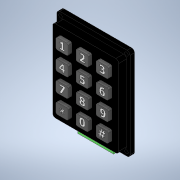
# Autodesk Inventor part: 3x4 Keypad
Saved by Autodesk Inventor 2020.2 (Build 242310000, 310)
## iProperties
Created: 2020-04-19
Part Number: 3x4 Keypad
Material: Generic
Document SubType Name: Modeling
Designer: Hayder_PC
Density: 1 g/cm^3
Appearance: Default
Author: Hayder_PC
Autodesk Inventor part; units mm, degrees
ref_plane "YZ Plane" through (0, 0, 0) normal (1, 0, 0) x (0, 1, 0)
ref_plane "XZ Plane" through (0, 0, 0) normal (0, 1, 0) x (-1, 0, 0)
sketch "Sketch1" plane through (0, 0, 0) normal (0, 0, 1) x (1, 0, 0)
  line L0 (-23.5, -32) -> (23.5, -32)
  line L1 (25.5, -30) -> (25.5, 30)
  line L2 (23.5, 32) -> (-23.5, 32)
  line L3 (-25.5, 30) -> (-25.5, -30)
  line L4 (-25.5, -32) -> (25.5, 32) construction
  line L5 (25.5, -32) -> (-25.5, 32) construction
  arc A0 (-23.5, 32) -> (-25.5, 30) centre (-23.5, 30) ccw
  arc A1 (25.5, 30) -> (23.5, 32) centre (23.5, 30) ccw
  arc A2 (23.5, -32) -> (25.5, -30) centre (23.5, -30) ccw
  arc A3 (-25.5, -30) -> (-23.5, -32) centre (-23.5, -30) ccw
  point P0 (0, 0)
  point P1 (-23, 29.5)
  point P2 (23, 29.5)
  point P3 (23, -29.5)
  point P4 (-23, -29.5)
  dimension "d0" = 64
  dimension "d1" = 51
  dimension "d7" = 2
  dimension "d26" = 2.5
  dimension "d27" = 2.5
  dimension "d28" = 46
  dimension "d29" = 59
  constraints: 12 end point, 8 point on circle, 8 point on line, 8 tangent, 4 centre point, 3 equal radius, 2 midpoint, 2 parallel, 2 vertical alignment, 1 horizontal, 1 horizontal alignment, 1 perpendicular
  measures "d0" distance of L5.start L4.end
  measures "d1" distance of L4.end L5.end
  measures "d7" radius of A0
  measures "d26" distance from line of L3 point (-23, 29.5)
  measures "d27" distance from line of L2 point (-23, 29.5)
  measures "d28" distance of point (23, 29.5) point (-23, 29.5)
  measures "d29" distance of point (23, -29.5) point (23, 29.5)
extrude "Extrusion1" add sketch "Sketch1" along normal blind 3.1
sketch "Sketch2" plane through (0, 0, 3.1) normal (0, 0, 1) x (1, 0, 0)
  line L0 (-23.5, -32) -> (23.5, -32) projected
  line L1 (25.5, -30) -> (25.5, 30) projected
  line L2 (23.5, 32) -> (-23.5, 32) projected
  line L3 (-25.5, 30) -> (-25.5, -30) projected
  line L4 (-21, -28.5) -> (21, -28.5)
  line L5 (23, -26.5) -> (23, 26.5)
  line L6 (21, 28.5) -> (-21, 28.5)
  line L7 (-23, 26.5) -> (-23, -26.5)
  line L8 (-23, -28.5) -> (23, 28.5) construction
  line L9 (23, -28.5) -> (-23, 28.5) construction
  arc A0 (-21, 28.5) -> (-23, 26.5) centre (-21, 26.5) ccw
  arc A1 (23, 26.5) -> (21, 28.5) centre (21, 26.5) ccw
  arc A2 (-23, -26.5) -> (-21, -28.5) centre (-21, -26.5) ccw
  arc A3 (21, -28.5) -> (23, -26.5) centre (21, -26.5) ccw
  arc A4 (-25.5, -30) -> (-23.5, -32) centre (-23.5, -30) ccw projected
  arc A5 (23.5, -32) -> (25.5, -30) centre (23.5, -30) ccw projected
  arc A6 (25.5, 30) -> (23.5, 32) centre (23.5, 30) ccw projected
  arc A7 (-23.5, 32) -> (-25.5, 30) centre (-23.5, 30) ccw projected
  point P0 (0, 0)
  dimension "d4" = 46
  dimension "d5" = 57
  dimension "d6" = 2
  constraints: 12 end point, 8 point on circle, 8 point on line, 8 tangent, 4 centre point, 3 equal radius, 2 midpoint, 2 parallel, 1 horizontal, 1 perpendicular
  measures "d4" distance of L8.end L9.end
  measures "d5" distance of L9.start L8.end
  measures "d6" radius of A0
extrude "Extrusion2" add sketch "Sketch2" along normal blind 5.4 contours A2 L7 A0 L6 A1 L5 A3 L4
sketch "Sketch3" plane through (0, 0, 8.5) normal (0, 0, 1) x (1, 0, 0)
  arc A0 (21, -28.5) -> (23, -26.5) centre (21, -26.5) ccw projected
  line L0 (23, -26.5) -> (23, 26.5) projected
  arc A1 (23, 26.5) -> (21, 28.5) centre (21, 26.5) ccw projected
  line L1 (21, 28.5) -> (-21, 28.5) projected
  arc A2 (-21, 28.5) -> (-23, 26.5) centre (-21, 26.5) ccw projected
  line L2 (-23, 26.5) -> (-23, -26.5) projected
  arc A3 (-23, -26.5) -> (-21, -28.5) centre (-21, -26.5) ccw projected
  line L3 (-21, -28.5) -> (21, -28.5) projected
  line L4 (10.75, 15.75) -> (17.25, 15.75)
  line L5 (18.25, 16.75) -> (18.25, 22.25)
  line L6 (17.25, 23.25) -> (10.75, 23.25)
  line L7 (9.75, 22.25) -> (9.75, 16.75)
  line L8 (9.75, 15.75) -> (18.25, 23.25) construction
  line L9 (18.25, 15.75) -> (9.75, 23.25) construction
  arc A4 (10.75, 23.25) -> (9.75, 22.25) centre (10.75, 22.25) ccw
  arc A5 (18.25, 22.25) -> (17.25, 23.25) centre (17.25, 22.25) ccw
  arc A6 (17.25, 15.75) -> (18.25, 16.75) centre (17.25, 16.75) ccw
  arc A7 (9.75, 16.75) -> (10.75, 15.75) centre (10.75, 16.75) ccw
  line L10 (-4.25, 22.25) -> (-4.25, 16.75)
  arc A8 (-4.25, 16.75) -> (-3.25, 15.75) centre (-3.25, 16.75) ccw
  arc A9 (-3.25, 23.25) -> (-4.25, 22.25) centre (-3.25, 22.25) ccw
  line L11 (-3.25, 15.75) -> (3.25, 15.75)
  line L12 (-4.25, 15.75) -> (4.25, 23.25) construction
  line L13 (4.25, 15.75) -> (-4.25, 23.25) construction
  arc A10 (3.25, 15.75) -> (4.25, 16.75) centre (3.25, 16.75) ccw
  line L14 (4.25, 16.75) -> (4.25, 22.25)
  line L15 (3.25, 23.25) -> (-3.25, 23.25)
  arc A11 (4.25, 22.25) -> (3.25, 23.25) centre (3.25, 22.25) ccw
  line L16 (-18.25, 22.25) -> (-18.25, 16.75)
  arc A12 (-18.25, 16.75) -> (-17.25, 15.75) centre (-17.25, 16.75) ccw
  arc A13 (-17.25, 23.25) -> (-18.25, 22.25) centre (-17.25, 22.25) ccw
  line L17 (-17.25, 15.75) -> (-10.75, 15.75)
  line L18 (-18.25, 15.75) -> (-9.75, 23.25) construction
  line L19 (-9.75, 15.75) -> (-18.25, 23.25) construction
  arc A14 (-10.75, 15.75) -> (-9.75, 16.75) centre (-10.75, 16.75) ccw
  line L20 (-9.75, 16.75) -> (-9.75, 22.25)
  line L21 (-10.75, 23.25) -> (-17.25, 23.25)
  arc A15 (-9.75, 22.25) -> (-10.75, 23.25) centre (-10.75, 22.25) ccw
  line L22 (9.75, 9.25) -> (9.75, 3.75)
  arc A16 (9.75, 3.75) -> (10.75, 2.75) centre (10.75, 3.75) ccw
  arc A17 (10.75, 10.25) -> (9.75, 9.25) centre (10.75, 9.25) ccw
  line L23 (10.75, 2.75) -> (17.25, 2.75)
  line L24 (9.75, 2.75) -> (18.25, 10.25) construction
  line L25 (18.25, 2.75) -> (9.75, 10.25) construction
  arc A18 (17.25, 2.75) -> (18.25, 3.75) centre (17.25, 3.75) ccw
  line L26 (18.25, 3.75) -> (18.25, 9.25)
  line L27 (17.25, 10.25) -> (10.75, 10.25)
  arc A19 (18.25, 9.25) -> (17.25, 10.25) centre (17.25, 9.25) ccw
  line L28 (-4.25, 9.25) -> (-4.25, 3.75)
  arc A20 (-4.25, 3.75) -> (-3.25, 2.75) centre (-3.25, 3.75) ccw
  arc A21 (-3.25, 10.25) -> (-4.25, 9.25) centre (-3.25, 9.25) ccw
  line L29 (-3.25, 2.75) -> (3.25, 2.75)
  line L30 (-4.25, 2.75) -> (4.25, 10.25) construction
  line L31 (4.25, 2.75) -> (-4.25, 10.25) construction
  arc A22 (3.25, 2.75) -> (4.25, 3.75) centre (3.25, 3.75) ccw
  line L32 (4.25, 3.75) -> (4.25, 9.25)
  line L33 (3.25, 10.25) -> (-3.25, 10.25)
  arc A23 (4.25, 9.25) -> (3.25, 10.25) centre (3.25, 9.25) ccw
  line L34 (-18.25, 9.25) -> (-18.25, 3.75)
  arc A24 (-18.25, 3.75) -> (-17.25, 2.75) centre (-17.25, 3.75) ccw
  arc A25 (-17.25, 10.25) -> (-18.25, 9.25) centre (-17.25, 9.25) ccw
  line L35 (-17.25, 2.75) -> (-10.75, 2.75)
  line L36 (-18.25, 2.75) -> (-9.75, 10.25) construction
  line L37 (-9.75, 2.75) -> (-18.25, 10.25) construction
  arc A26 (-10.75, 2.75) -> (-9.75, 3.75) centre (-10.75, 3.75) ccw
  line L38 (-9.75, 3.75) -> (-9.75, 9.25)
  line L39 (-10.75, 10.25) -> (-17.25, 10.25)
  arc A27 (-9.75, 9.25) -> (-10.75, 10.25) centre (-10.75, 9.25) ccw
  line L40 (9.75, -3.75) -> (9.75, -9.25)
  arc A28 (9.75, -9.25) -> (10.75, -10.25) centre (10.75, -9.25) ccw
  arc A29 (10.75, -2.75) -> (9.75, -3.75) centre (10.75, -3.75) ccw
  line L41 (10.75, -10.25) -> (17.25, -10.25)
  line L42 (9.75, -10.25) -> (18.25, -2.75) construction
  line L43 (18.25, -10.25) -> (9.75, -2.75) construction
  arc A30 (17.25, -10.25) -> (18.25, -9.25) centre (17.25, -9.25) ccw
  line L44 (18.25, -9.25) -> (18.25, -3.75)
  line L45 (17.25, -2.75) -> (10.75, -2.75)
  arc A31 (18.25, -3.75) -> (17.25, -2.75) centre (17.25, -3.75) ccw
  line L46 (-4.25, -3.75) -> (-4.25, -9.25)
  arc A32 (-4.25, -9.25) -> (-3.25, -10.25) centre (-3.25, -9.25) ccw
  arc A33 (-3.25, -2.75) -> (-4.25, -3.75) centre (-3.25, -3.75) ccw
  line L47 (-3.25, -10.25) -> (3.25, -10.25)
  line L48 (-4.25, -10.25) -> (4.25, -2.75) construction
  line L49 (4.25, -10.25) -> (-4.25, -2.75) construction
  arc A34 (3.25, -10.25) -> (4.25, -9.25) centre (3.25, -9.25) ccw
  line L50 (4.25, -9.25) -> (4.25, -3.75)
  line L51 (3.25, -2.75) -> (-3.25, -2.75)
  arc A35 (4.25, -3.75) -> (3.25, -2.75) centre (3.25, -3.75) ccw
  line L52 (-18.25, -3.75) -> (-18.25, -9.25)
  arc A36 (-18.25, -9.25) -> (-17.25, -10.25) centre (-17.25, -9.25) ccw
  arc A37 (-17.25, -2.75) -> (-18.25, -3.75) centre (-17.25, -3.75) ccw
  line L53 (-17.25, -10.25) -> (-10.75, -10.25)
  line L54 (-18.25, -10.25) -> (-9.75, -2.75) construction
  line L55 (-9.75, -10.25) -> (-18.25, -2.75) construction
  arc A38 (-10.75, -10.25) -> (-9.75, -9.25) centre (-10.75, -9.25) ccw
  line L56 (-9.75, -9.25) -> (-9.75, -3.75)
  line L57 (-10.75, -2.75) -> (-17.25, -2.75)
  arc A39 (-9.75, -3.75) -> (-10.75, -2.75) centre (-10.75, -3.75) ccw
  line L58 (9.75, -16.75) -> (9.75, -22.25)
  arc A40 (9.75, -22.25) -> (10.75, -23.25) centre (10.75, -22.25) ccw
  arc A41 (10.75, -15.75) -> (9.75, -16.75) centre (10.75, -16.75) ccw
  line L59 (10.75, -23.25) -> (17.25, -23.25)
  line L60 (9.75, -23.25) -> (18.25, -15.75) construction
  line L61 (18.25, -23.25) -> (9.75, -15.75) construction
  arc A42 (17.25, -23.25) -> (18.25, -22.25) centre (17.25, -22.25) ccw
  line L62 (18.25, -22.25) -> (18.25, -16.75)
  line L63 (17.25, -15.75) -> (10.75, -15.75)
  arc A43 (18.25, -16.75) -> (17.25, -15.75) centre (17.25, -16.75) ccw
  line L64 (-4.25, -16.75) -> (-4.25, -22.25)
  arc A44 (-4.25, -22.25) -> (-3.25, -23.25) centre (-3.25, -22.25) ccw
  arc A45 (-3.25, -15.75) -> (-4.25, -16.75) centre (-3.25, -16.75) ccw
  line L65 (-3.25, -23.25) -> (3.25, -23.25)
  line L66 (-4.25, -23.25) -> (4.25, -15.75) construction
  line L67 (4.25, -23.25) -> (-4.25, -15.75) construction
  arc A46 (3.25, -23.25) -> (4.25, -22.25) centre (3.25, -22.25) ccw
  line L68 (4.25, -22.25) -> (4.25, -16.75)
  line L69 (3.25, -15.75) -> (-3.25, -15.75)
  arc A47 (4.25, -16.75) -> (3.25, -15.75) centre (3.25, -16.75) ccw
  line L70 (-18.25, -16.75) -> (-18.25, -22.25)
  arc A48 (-18.25, -22.25) -> (-17.25, -23.25) centre (-17.25, -22.25) ccw
  arc A49 (-17.25, -15.75) -> (-18.25, -16.75) centre (-17.25, -16.75) ccw
  line L71 (-17.25, -23.25) -> (-10.75, -23.25)
  line L72 (-18.25, -23.25) -> (-9.75, -15.75) construction
  line L73 (-9.75, -23.25) -> (-18.25, -15.75) construction
  arc A50 (-10.75, -23.25) -> (-9.75, -22.25) centre (-10.75, -22.25) ccw
  line L74 (-9.75, -22.25) -> (-9.75, -16.75)
  line L75 (-10.75, -15.75) -> (-17.25, -15.75)
  arc A51 (-9.75, -16.75) -> (-10.75, -15.75) centre (-10.75, -16.75) ccw
  point P0 (0, 0)
  point P1 (14, 19.5)
  point P2 (0, 19.5)
  point P3 (-14, 19.5)
  point P4 (14, 6.5)
  point P5 (0, 6.5)
  point P6 (-14, 6.5)
  point P7 (14, -6.5)
  point P8 (0, -6.5)
  point P9 (-14, -6.5)
  point P10 (14, -19.5)
  point P11 (0, -19.5)
  point P12 (-14, -19.5)
  dimension "d10" = 8.5
  dimension "d11" = 7.5
  dimension "d12" = 1
  dimension "d15" = 9
  dimension "d18" = 14
  dimension "d21" = 13
  constraints: 144 end point, 96 point on circle, 96 point on line, 48 centre point, 24 midpoint, 8 tangent, 3 equal radius, 2 collinear, 2 horizontal, 2 parallel, 1 perpendicular, 1 vertical, 295 other
  measures "d10" distance of L8.end L9.end
  measures "d11" distance of L9.start L8.end
  measures "d12" radius of A4
  measures "d15" distance from line of L0 point (14, 19.5)
  measures "d18" distance of L8.start L12.start
  measures "d21" distance of L8.start L24.start
extrude "Extrusion3" add sketch "Sketch3" along normal blind 2.5 contours A7 L7 A4 L6 A5 L5 A6 L4 | A9 L15 A11 L14 A10 L11 A8 L10 | A13 L21 A15 L20 A14 L17 A12 L16 | A17 L27 A19 L26 A18 L23 A16 L22 | A21 L33 A23 L32 A22 L29 A20 L28 | A25 L39 A27 L38 A26 L35 A24 L34 | A29 L45 A31 L44 A30 L41 A28 L40 | A33 L51 A35 L50 A34 L47 A32 L46 | A37 L57 A39 L56 A38 L53 A36 L52 | A41 L63 A43 L62 A42 L59 A40 L58 | A45 L69 A47 L68 A46 L65 A44 L64 | A49 L75 A51 L74 A50 L71 A48 L70
sketch "Sketch4" plane through (0, 0, 3.1) normal (0, 0, 1) x (1, 0, 0)
  line L0 (-21, 28.5) -> (21, 28.5) projected
  arc A0 (23, 26.5) -> (21, 28.5) centre (21, 26.5) ccw projected
  line L1 (23, 26.5) -> (23, -26.5) projected
  arc A1 (21, -28.5) -> (23, -26.5) centre (21, -26.5) ccw projected
  line L2 (21, -28.5) -> (-21, -28.5) projected
  arc A2 (-23, -26.5) -> (-21, -28.5) centre (-21, -26.5) ccw projected
  line L3 (-23, -26.5) -> (-23, 26.5) projected
  arc A3 (-21, 28.5) -> (-23, 26.5) centre (-21, 26.5) ccw projected
  line L4 (-23.5, -32) -> (23.5, -32) projected
  arc A4 (23.5, -32) -> (25.5, -30) centre (23.5, -30) ccw projected
  line L5 (25.5, -30) -> (25.5, 30) projected
  arc A5 (25.5, 30) -> (23.5, 32) centre (23.5, 30) ccw projected
  line L6 (23.5, 32) -> (-23.5, 32) projected
  arc A6 (-23.5, 32) -> (-25.5, 30) centre (-23.5, 30) ccw projected
  line L7 (-25.5, 30) -> (-25.5, -30) projected
  arc A7 (-25.5, -30) -> (-23.5, -32) centre (-23.5, -30) ccw projected
  point P0 (0, 0)
  point P1 (-23, 29.5)
  point P2 (23, 29.5)
  point P3 (23, -29.5)
  point P4 (-23, -29.5)
  dimension "d30" = 2.5
  dimension "d31" = 2.5
  dimension "d32" = 46
  dimension "d33" = 59
  constraints: 2 horizontal alignment, 2 vertical alignment
  measures "d30" distance from line of L6 point (-23, 29.5)
  measures "d31" distance from line of L7 point (-23, 29.5)
  measures "d32" distance of point (23, 29.5) point (-23, 29.5)
  measures "d33" distance of point (23, -29.5) point (23, 29.5)
hole "Hole1" at (-23, 29.5, 3.1) at (23, 29.5, 3.1) at (23, -29.5, 3.1) at (-23, -29.5, 3.1) direction (0, 0, -1) diameter 2.4 end through all
ref_plane "Work Plane2" through (0, 0, 1.5) normal (0, 0, 1) x (1, 0, 0)
sketch "Sketch8" plane through (0, 0, 1.5) normal (0, 0, 1) x (1, 0, 0)
  line L0 (-23.5, -32) -> (23.5, -32) projected
  line L1 (-12.5, -32) -> (12.5, -32)
  line L2 (12.5, -32) -> (12.5, -37)
  line L3 (12.5, -37) -> (-12.5, -37)
  line L4 (-12.5, -37) -> (-12.5, -32)
  line L5 (-25.5, 30) -> (-25.5, -30) projected
  point P0 (0, 0)
  point P1 (12.5, -32)
  dimension "d60" = 25
  dimension "d61" = 5
  dimension "d62" = 13
  constraints: 8 end point, 2 parallel, 1 horizontal, 1 perpendicular, 1 point on line
  measures "d60" distance of L2.end L3.end
  measures "d61" distance of L1.end L2.end
  measures "d62" distance between parallel lines of L5 L4
extrude "Extrusion6" add sketch "Sketch8" against normal blind 1
sketch "Sketch9" plane through (0, 0, 1.5) normal (0, 0, 1) x (1, 0, 0)
  circle A0 centre (-8.75, -34.5) radius 0.5
  line L0 (-12.5, -32) -> (-12.5, -37) projected
  line L1 (-12.5, -37) -> (12.5, -37) projected
  line L2 (-8.75, -34.5) -> (7.0736, -34.5) construction
  line L3 (-6.25, -34.5) -> (9.5736, -34.5) construction
  circle A1 centre (-6.25, -34.5) radius 0.5
  line L4 (-3.75, -34.5) -> (12.0736, -34.5) construction
  circle A2 centre (-3.75, -34.5) radius 0.5
  line L5 (-1.25, -34.5) -> (14.5736, -34.5) construction
  circle A3 centre (-1.25, -34.5) radius 0.5
  line L6 (1.25, -34.5) -> (17.0736, -34.5) construction
  circle A4 centre (1.25, -34.5) radius 0.5
  line L7 (3.75, -34.5) -> (19.5736, -34.5) construction
  circle A5 centre (3.75, -34.5) radius 0.5
  line L8 (6.25, -34.5) -> (22.0736, -34.5) construction
  circle A6 centre (6.25, -34.5) radius 0.5
  line L9 (8.75, -34.5) -> (24.5736, -34.5) construction
  circle A7 centre (8.75, -34.5) radius 0.5
  point P0 (0, 0)
  dimension "d65" = 1
  dimension "d66" = 3.75
  dimension "d67" = 2.5
  dimension "d70" = 2.5
  constraints: 16 end point, 8 centre point, 2 horizontal, 1 collinear, 27 other
  measures "d65" diameter of A0
  measures "d66" distance from line of L0 L2.start
  measures "d67" distance from line of L1 L2.start
  measures "d70" distance of L2.start L3.start
extrude "Extrusion7" cut sketch "Sketch9" against normal blind 1
sketch "Sketch11" plane through (0, 0, 11) normal (0, 0, 1) x (1, 0, 0)
  line L0 (-16.2137, 22.189) -> (-9.5825, 22.189) construction
  line L1 (-9.5825, 22.189) -> (-9.5825, 17.2629) construction
  line L2 (-9.5825, 17.2629) -> (-16.2137, 17.2629) construction
  line L3 (-16.2137, 17.2629) -> (-16.2137, 22.189) construction
  line L4 (-2.1702, 22.189) -> (4.461, 22.189) construction
  line L5 (4.461, 22.189) -> (4.461, 17.2629) construction
  line L6 (4.461, 17.2629) -> (-2.1702, 17.2629) construction
  line L7 (-2.1702, 17.2629) -> (-2.1702, 22.189) construction
  line L8 (11.6989, 22.189) -> (18.3301, 22.189) construction
  line L9 (18.3301, 22.189) -> (18.3301, 17.2629) construction
  line L10 (18.3301, 17.2629) -> (11.6989, 17.2629) construction
  line L11 (11.6989, 17.2629) -> (11.6989, 22.189) construction
  line L12 (-16.2137, 8.9305) -> (-9.5825, 8.9305) construction
  line L13 (-9.5825, 8.9305) -> (-9.5825, 4.0044) construction
  line L14 (-9.5825, 4.0044) -> (-16.2137, 4.0044) construction
  line L15 (-16.2137, 4.0044) -> (-16.2137, 8.9305) construction
  line L16 (-2.1702, 8.9305) -> (4.461, 8.9305) construction
  line L17 (4.461, 8.9305) -> (4.461, 4.0044) construction
  line L18 (4.461, 4.0044) -> (-2.1702, 4.0044) construction
  line L19 (-2.1702, 4.0044) -> (-2.1702, 8.9305) construction
  line L20 (11.6989, 8.9305) -> (18.3301, 8.9305) construction
  line L21 (18.3301, 8.9305) -> (18.3301, 4.0044) construction
  line L22 (18.3301, 4.0044) -> (11.6989, 4.0044) construction
  line L23 (11.6989, 4.0044) -> (11.6989, 8.9305) construction
  line L24 (-16.2137, -4.0005) -> (-9.5825, -4.0005) construction
  line L25 (-9.5825, -4.0005) -> (-9.5825, -8.9266) construction
  line L26 (-9.5825, -8.9266) -> (-16.2137, -8.9266) construction
  line L27 (-16.2137, -8.9266) -> (-16.2137, -4.0005) construction
  line L28 (-2.1702, -4.0005) -> (4.461, -4.0005) construction
  line L29 (4.461, -4.0005) -> (4.461, -8.9266) construction
  line L30 (4.461, -8.9266) -> (-2.1702, -8.9266) construction
  line L31 (-2.1702, -8.9266) -> (-2.1702, -4.0005) construction
  line L32 (12.2001, -4.0005) -> (18.8313, -4.0005) construction
  line L33 (18.8313, -4.0005) -> (18.8313, -8.9266) construction
  line L34 (18.8313, -8.9266) -> (12.2001, -8.9266) construction
  line L35 (12.2001, -8.9266) -> (12.2001, -4.0005) construction
  line L36 (10.8904, -16.8079) -> (17.5216, -16.8079) construction
  line L37 (17.5216, -16.8079) -> (17.5216, -21.734) construction
  line L38 (17.5216, -21.734) -> (10.8904, -21.734) construction
  line L39 (10.8904, -21.734) -> (10.8904, -16.8079) construction
  line L40 (-2.1702, -16.6356) -> (4.461, -16.6356) construction
  line L41 (4.461, -16.6356) -> (4.461, -21.5617) construction
  line L42 (4.461, -21.5617) -> (-2.1702, -21.5617) construction
  line L43 (-2.1702, -21.5617) -> (-2.1702, -16.6356) construction
  line L44 (-16.1103, -17.8074) -> (-9.4791, -17.8074) construction
  line L45 (-9.4791, -17.8074) -> (-9.4791, -22.7335) construction
  line L46 (-9.4791, -22.7335) -> (-16.1103, -22.7335) construction
  line L47 (-16.1103, -22.7335) -> (-16.1103, -17.8074) construction
  line L48 (-12.2551, 17.1769) -> (-15.5573, 17.1769)
  line L49 (-15.5573, 17.1769) -> (-15.5573, 18.048)
  line L50 (-15.5573, 18.048) -> (-14.5039, 18.048)
  line L51 (-14.5039, 18.048) -> (-14.5039, 20.6939)
  line L52 (-14.5039, 20.6939) -> (-15.5573, 20.6939)
  line L53 (-15.5573, 20.6939) -> (-15.5573, 21.5083)
  spline S0 degree 2 poles (-15.5573, 21.5083) (-15.3264, 21.5083) (-14.8685, 21.5691) (-14.7308, 21.6339) knots 0 0 0 1 2 2 2
  spline S1 degree 2 poles (-14.7308, 21.6339) (-14.5727, 21.7149) (-14.3944, 21.9864) (-14.3782, 22.189) knots 0 0 0 1 2 2 2
  line L54 (-14.3782, 22.189) -> (-13.2842, 22.189)
  line L55 (-13.2842, 22.189) -> (-13.2842, 18.048)
  line L56 (-13.2842, 18.048) -> (-12.2551, 18.048)
  line L57 (-12.2551, 18.048) -> (-12.2551, 17.1769)
  line L58 (2.0113, 17.0918) -> (-1.6637, 17.0918)
  line L59 (-1.6637, 17.0918) -> (-1.6637, 17.9062)
  spline S2 degree 2 poles (-1.6637, 17.9062) (-1.1978, 18.279) (-0.4522, 18.9354) (-0.1726, 19.2311) knots 0 0 0 1 2 2 2
  spline S3 degree 2 poles (-0.1726, 19.2311) (0.1961, 19.6161) (0.5243, 20.2036) (0.5243, 20.5115) knots 0 0 0 1 2 2 2
  spline S4 degree 2 poles (0.5243, 20.5115) (0.5243, 20.86) (0.1069, 21.2328) (-0.2658, 21.2328) knots 0 0 0 1 2 2 2
  spline S5 degree 2 poles (-0.2658, 21.2328) (-0.4563, 21.2328) (-0.7966, 21.1396) (-0.9709, 21.0666) knots 0 0 0 1 2 2 2
  spline S6 degree 2 poles (-0.9709, 21.0666) (-1.141, 20.9897) (-1.3842, 20.8276) (-1.4449, 20.7871) knots 0 0 0 1 2 2 2
  line L60 (-1.4449, 20.7871) -> (-1.5422, 20.7871)
  line L61 (-1.5422, 20.7871) -> (-1.5422, 21.877)
  spline S7 degree 2 poles (-1.5422, 21.877) (-1.3315, 21.9783) (-0.432, 22.189) (-0.0146, 22.189) knots 0 0 0 1 2 2 2
  spline S8 degree 2 poles (-0.0146, 22.189) (0.8768, 22.189) (1.7925, 21.3948) (1.7925, 20.6777) knots 0 0 0 1 2 2 2
  spline S9 degree 2 poles (1.7925, 20.6777) (1.7925, 20.236) (1.3752, 19.3851) (0.893, 18.8989) knots 0 0 0 1 2 2 2
  spline S10 degree 2 poles (0.893, 18.8989) (0.5891, 18.5991) (0.0178, 18.1331) (-0.1078, 18.0358) knots 0 0 0 1 2 2 2
  line L62 (-0.1078, 18.0358) -> (2.0113, 18.0358)
  line L63 (2.0113, 18.0358) -> (2.0113, 17.0918)
  line L64 (-12.3056, -20.1412) -> (-12.6501, -20.6518)
  line L65 (-12.6501, -20.6518) -> (-13.6995, -19.9387)
  line L66 (-13.6995, -19.9387) -> (-13.663, -21.1056)
  line L67 (-13.663, -21.1056) -> (-14.3356, -21.1056)
  line L68 (-14.3356, -21.1056) -> (-14.3154, -19.9711)
  line L69 (-14.3154, -19.9711) -> (-15.3405, -20.6558)
  line L70 (-15.3405, -20.6558) -> (-15.6849, -20.1372)
  line L71 (-15.6849, -20.1372) -> (-14.5261, -19.4565)
  line L72 (-14.5261, -19.4565) -> (-15.6768, -18.7677)
  line L73 (-15.6768, -18.7677) -> (-15.3405, -18.249)
  line L74 (-15.3405, -18.249) -> (-14.3154, -18.9459)
  line L75 (-14.3154, -18.9459) -> (-14.3356, -17.8074)
  line L76 (-14.3356, -17.8074) -> (-13.6671, -17.8074)
  line L77 (-13.6671, -17.8074) -> (-13.6873, -18.9459)
  line L78 (-13.6873, -18.9459) -> (-12.6501, -18.2531)
  line L79 (-12.6501, -18.2531) -> (-12.3056, -18.7717)
  line L80 (-12.3056, -18.7717) -> (-13.4685, -19.4524)
  line L81 (-13.4685, -19.4524) -> (-12.3056, -20.1412)
  spline S11 degree 2 poles (1.9465, -19.2369) (1.9465, -19.8852) (1.7398, -20.8576) (1.5089, -21.1858) knots 0 0 0 1 2 2 2
  spline S12 degree 2 poles (1.5089, -21.1858) (1.282, -21.51) (0.5486, -21.8423) (0.0218, -21.8423) knots 0 0 0 1 2 2 2
  spline S13 degree 2 poles (0.0218, -21.8423) (-0.5089, -21.8423) (-1.2383, -21.51) (-1.4692, -21.1777) knots 0 0 0 1 2 2 2
  spline S14 degree 2 poles (-1.4692, -21.1777) (-1.7002, -20.8495) (-1.9068, -19.8852) (-1.9068, -19.2369) knots 0 0 0 1 2 2 2
  spline S15 degree 2 poles (-1.9068, -19.2369) (-1.9068, -18.5724) (-1.7002, -17.6324) (-1.4652, -17.292) knots 0 0 0 1 2 2 2
  spline S16 degree 2 poles (-1.4652, -17.292) (-1.2302, -16.9598) (-0.4887, -16.6356) (0.0218, -16.6356) knots 0 0 0 1 2 2 2
  spline S17 degree 2 poles (0.0218, -16.6356) (0.5607, -16.6356) (1.282, -16.976) (1.5129, -17.3123) knots 0 0 0 1 2 2 2
  spline S18 degree 2 poles (1.5129, -17.3123) (1.7398, -17.6405) (1.9465, -18.6089) (1.9465, -19.2369) knots 0 0 0 1 2 2 2
  spline S19 degree 2 poles (0.6864, -19.2369) (0.6864, -18.309) (0.3825, -17.5594) (0.0218, -17.5594) knots 0 0 0 1 2 2 2
  spline S20 degree 2 poles (0.0218, -17.5594) (-0.3388, -17.5594) (-0.6467, -18.309) (-0.6467, -19.241) knots 0 0 0 1 2 2 2
  spline S21 degree 2 poles (-0.6467, -19.241) (-0.6467, -20.1567) (-0.3388, -20.9184) (0.0218, -20.9184) knots 0 0 0 1 2 2 2
  spline S22 degree 2 poles (0.0218, -20.9184) (0.3784, -20.9184) (0.6864, -20.1567) (0.6864, -19.2369) knots 0 0 0 1 2 2 2
  line L82 (16.1011, -18.7447) -> (15.076, -18.7447)
  line L83 (15.076, -18.7447) -> (14.8045, -19.8428)
  line L84 (14.8045, -19.8428) -> (15.7122, -19.8428)
  line L85 (15.7122, -19.8428) -> (15.7122, -20.6167)
  line L86 (15.7122, -20.6167) -> (14.606, -20.6167)
  line L87 (14.606, -20.6167) -> (14.3062, -21.8079)
  line L88 (14.3062, -21.8079) -> (13.5282, -21.8079)
  line L89 (13.5282, -21.8079) -> (13.828, -20.6167)
  line L90 (13.828, -20.6167) -> (12.965, -20.6167)
  line L91 (12.965, -20.6167) -> (12.6652, -21.8079)
  line L92 (12.6652, -21.8079) -> (11.8791, -21.8079)
  line L93 (11.8791, -21.8079) -> (12.1789, -20.6167)
  line L94 (12.1789, -20.6167) -> (11.3078, -20.6167)
  line L95 (11.3078, -20.6167) -> (11.3078, -19.8428)
  line L96 (11.3078, -19.8428) -> (12.3734, -19.8428)
  line L97 (12.3734, -19.8428) -> (12.6449, -18.7447)
  line L98 (12.6449, -18.7447) -> (11.7008, -18.7447)
  line L99 (11.7008, -18.7447) -> (11.7008, -17.9708)
  line L100 (11.7008, -17.9708) -> (12.8394, -17.9708)
  line L101 (12.8394, -17.9708) -> (13.1311, -16.8079)
  line L102 (13.1311, -16.8079) -> (13.9212, -16.8079)
  line L103 (13.9212, -16.8079) -> (13.6295, -17.9708)
  line L104 (13.6295, -17.9708) -> (14.4885, -17.9708)
  line L105 (14.4885, -17.9708) -> (14.7802, -16.8079)
  line L106 (14.7802, -16.8079) -> (15.5704, -16.8079)
  line L107 (15.5704, -16.8079) -> (15.2746, -17.9708)
  line L108 (15.2746, -17.9708) -> (16.1011, -17.9708)
  line L109 (16.1011, -17.9708) -> (16.1011, -18.7447)
  line L110 (14.3062, -18.7366) -> (13.4269, -18.7366)
  line L111 (13.4269, -18.7366) -> (13.1473, -19.8509)
  line L112 (13.1473, -19.8509) -> (14.0266, -19.8509)
  line L113 (14.0266, -19.8509) -> (14.3062, -18.7366)
  spline S23 degree 2 poles (16.2519, -6.3222) (16.2519, -6.9584) (15.9561, -8.02) (15.6442, -8.4008) knots 0 0 0 1 2 2 2
  spline S24 degree 2 poles (15.6442, -8.4008) (15.32, -8.7858) (14.3638, -9.1991) (13.6668, -9.1991) knots 0 0 0 1 2 2 2
  spline S25 degree 2 poles (13.6668, -9.1991) (13.4318, -9.1991) (12.9213, -9.1383) (12.8362, -9.114) knots 0 0 0 1 2 2 2
  line L114 (12.8362, -9.114) -> (12.8362, -8.1334)
  line L115 (12.8362, -8.1334) -> (12.9335, -8.1334)
  spline S26 degree 2 poles (12.9335, -8.1334) (13.0267, -8.182) (13.3751, -8.2874) (13.679, -8.2874) knots 0 0 0 1 2 2 2
  spline S27 degree 2 poles (13.679, -8.2874) (13.9262, -8.2874) (14.384, -8.1577) (14.5461, -8.0159) knots 0 0 0 1 2 2 2
  spline S28 degree 2 poles (14.5461, -8.0159) (14.7203, -7.866) (14.9472, -7.4243) (14.9878, -7.0921) knots 0 0 0 1 2 2 2
  spline S29 degree 2 poles (14.9878, -7.0921) (14.7203, -7.2582) (14.2584, -7.4365) (13.914, -7.4365) knots 0 0 0 1 2 2 2
  spline S30 degree 2 poles (13.914, -7.4365) (13.6587, -7.4365) (13.1847, -7.2987) (12.9902, -7.1529) knots 0 0 0 1 2 2 2
  spline S31 degree 2 poles (12.9902, -7.1529) (12.7309, -6.9543) (12.427, -6.3182) (12.427, -5.8158) knots 0 0 0 1 2 2 2
  spline S32 degree 2 poles (12.427, -5.8158) (12.427, -5.4227) (12.6944, -4.7623) (12.9375, -4.5192) knots 0 0 0 1 2 2 2
  spline S33 degree 2 poles (12.9375, -4.5192) (13.1806, -4.276) (13.8856, -4.0005) (14.3192, -4.0005) knots 0 0 0 1 2 2 2
  spline S34 degree 2 poles (14.3192, -4.0005) (14.7568, -4.0005) (15.4335, -4.2436) (15.6766, -4.4989) knots 0 0 0 1 2 2 2
  spline S35 degree 2 poles (15.6766, -4.4989) (15.9602, -4.7825) (16.2519, -5.682) (16.2519, -6.3222) knots 0 0 0 1 2 2 2
  spline S36 degree 2 poles (15.008, -6.1358) (15.008, -5.7266) (14.8702, -5.1999) (14.7446, -5.054) knots 0 0 0 1 2 2 2
  spline S37 degree 2 poles (14.7446, -5.054) (14.6596, -4.9446) (14.4408, -4.8514) (14.3151, -4.8514) knots 0 0 0 1 2 2 2
  spline S38 degree 2 poles (14.3151, -4.8514) (14.2017, -4.8514) (13.991, -4.9405) (13.8937, -5.054) knots 0 0 0 1 2 2 2
  spline S39 degree 2 poles (13.8937, -5.054) (13.8087, -5.1512) (13.6871, -5.5281) (13.6871, -5.7509) knots 0 0 0 1 2 2 2
  spline S40 degree 2 poles (13.6871, -5.7509) (13.6871, -5.994) (13.8127, -6.306) (13.9181, -6.3992) knots 0 0 0 1 2 2 2
  spline S41 degree 2 poles (13.9181, -6.3992) (14.0275, -6.4924) (14.2989, -6.5653) (14.4691, -6.5653) knots 0 0 0 1 2 2 2
  spline S42 degree 2 poles (14.4691, -6.5653) (14.6109, -6.5653) (14.9067, -6.4884) (14.9999, -6.4478) knots 0 0 0 1 2 2 2
  spline S43 degree 2 poles (14.9999, -6.4478) (14.9999, -6.4114) (15.008, -6.2736) (15.008, -6.1358) knots 0 0 0 1 2 2 2
  spline S44 degree 2 poles (1.9992, -7.7242) (1.9992, -8.0443) (1.7317, -8.5994) (1.4765, -8.802) knots 0 0 0 1 2 2 2
  spline S45 degree 2 poles (1.4765, -8.802) (1.2212, -9.0046) (0.4878, -9.2315) (0.0137, -9.2315) knots 0 0 0 1 2 2 2
  spline S46 degree 2 poles (0.0137, -9.2315) (-0.4927, -9.2315) (-1.2504, -9.0005) (-1.4936, -8.802) knots 0 0 0 1 2 2 2
  spline S47 degree 2 poles (-1.4936, -8.802) (-1.7326, -8.6034) (-1.9595, -8.0645) (-1.9595, -7.7647) knots 0 0 0 1 2 2 2
  spline S48 degree 2 poles (-1.9595, -7.7647) (-1.9595, -7.3352) (-1.4854, -6.7639) (-1.0357, -6.5735) knots 0 0 0 1 2 2 2
  line L116 (-1.0357, -6.5735) -> (-1.0357, -6.5532)
  spline S49 degree 2 poles (-1.0357, -6.5532) (-1.4773, -6.3384) (-1.8258, -5.7266) (-1.8258, -5.3498) knots 0 0 0 1 2 2 2
  spline S50 degree 2 poles (-1.8258, -5.3498) (-1.8258, -5.0743) (-1.5827, -4.5921) (-1.3436, -4.4017) knots 0 0 0 1 2 2 2
  spline S51 degree 2 poles (-1.3436, -4.4017) (-1.1127, -4.2193) (-0.4117, -4.0005) (0.0259, -4.0005) knots 0 0 0 1 2 2 2
  spline S52 degree 2 poles (0.0259, -4.0005) (0.4878, -4.0005) (1.1766, -4.1991) (1.3995, -4.3611) knots 0 0 0 1 2 2 2
  spline S53 degree 2 poles (1.3995, -4.3611) (1.6264, -4.5232) (1.8695, -4.9932) (1.8695, -5.2647) knots 0 0 0 1 2 2 2
  spline S54 degree 2 poles (1.8695, -5.2647) (1.8695, -5.6213) (1.4562, -6.1926) (1.0308, -6.3911) knots 0 0 0 1 2 2 2
  line L117 (1.0308, -6.3911) -> (1.0308, -6.4073)
  spline S55 degree 2 poles (1.0308, -6.4073) (1.5291, -6.6099) (1.9992, -7.2663) (1.9992, -7.7242) knots 0 0 0 1 2 2 2
  spline S56 degree 2 poles (0.7593, -7.7769) (0.7593, -7.5297) (0.5486, -7.2704) (0.2082, -7.1042) knots 0 0 0 1 2 2 2
  spline S57 degree 2 poles (0.2082, -7.1042) (0.111, -7.0597) (-0.2577, -6.9179) (-0.3995, -6.8571) knots 0 0 0 1 2 2 2
  spline S58 degree 2 poles (-0.3995, -6.8571) (-0.5292, -6.9867) (-0.7359, -7.3757) (-0.7359, -7.6067) knots 0 0 0 1 2 2 2
  spline S59 degree 2 poles (-0.7359, -7.6067) (-0.7359, -7.9551) (-0.2901, -8.3725) (0.0705, -8.3725) knots 0 0 0 1 2 2 2
  spline S60 degree 2 poles (0.0705, -8.3725) (0.1718, -8.3725) (0.423, -8.3076) (0.5202, -8.2428) knots 0 0 0 1 2 2 2
  spline S61 degree 2 poles (0.5202, -8.2428) (0.6296, -8.1658) (0.7593, -7.9551) (0.7593, -7.7769) knots 0 0 0 1 2 2 2
  spline S62 degree 2 poles (0.6499, -5.4106) (0.6499, -5.1553) (0.3136, -4.8514) (0.0259, -4.8514) knots 0 0 0 1 2 2 2
  spline S63 degree 2 poles (0.0259, -4.8514) (-0.2496, -4.8514) (-0.5859, -5.1269) (-0.5859, -5.3295) knots 0 0 0 1 2 2 2
  spline S64 degree 2 poles (-0.5859, -5.3295) (-0.5859, -5.5281) (-0.3833, -5.7752) (-0.1686, -5.8765) knots 0 0 0 1 2 2 2
  spline S65 degree 2 poles (-0.1686, -5.8765) (-0.0754, -5.9252) (0.1839, -6.0264) (0.3987, -6.1075) knots 0 0 0 1 2 2 2
  spline S66 degree 2 poles (0.3987, -6.1075) (0.5283, -5.9373) (0.6499, -5.6172) (0.6499, -5.4106) knots 0 0 0 1 2 2 2
  line L118 (-12.1416, -4.9932) -> (-14.2769, -9.0005)
  line L119 (-14.2769, -9.0005) -> (-15.6708, -9.0005)
  line L120 (-15.6708, -9.0005) -> (-13.4382, -4.9446)
  line L121 (-13.4382, -4.9446) -> (-15.8207, -4.9446)
  line L122 (-15.8207, -4.9446) -> (-15.8207, -4.0005)
  line L123 (-15.8207, -4.0005) -> (-12.1416, -4.0005)
  line L124 (-12.1416, -4.0005) -> (-12.1416, -4.9932)
  line L125 (-11.9714, 5.0975) -> (-12.6481, 5.0975)
  line L126 (-12.6481, 5.0975) -> (-12.6481, 3.9184)
  line L127 (-12.6481, 3.9184) -> (-13.8596, 3.9184)
  line L128 (-13.8596, 3.9184) -> (-13.8596, 5.0975)
  line L129 (-13.8596, 5.0975) -> (-16.0638, 5.0975)
  line L130 (-16.0638, 5.0975) -> (-16.0638, 6.0294)
  line L131 (-16.0638, 6.0294) -> (-13.9001, 8.9305)
  line L132 (-13.9001, 8.9305) -> (-12.6481, 8.9305)
  line L133 (-12.6481, 8.9305) -> (-12.6481, 5.997)
  line L134 (-12.6481, 5.997) -> (-11.9714, 5.997)
  line L135 (-11.9714, 5.997) -> (-11.9714, 5.0975)
  line L136 (-13.8596, 5.997) -> (-13.8596, 7.6988)
  line L137 (-13.8596, 7.6988) -> (-15.1278, 5.997)
  line L138 (-15.1278, 5.997) -> (-13.8596, 5.997)
  spline S67 degree 2 poles (1.8979, 5.6242) (1.8979, 5.2312) (1.6304, 4.5667) (1.3671, 4.3276) knots 0 0 0 1 2 2 2
  spline S68 degree 2 poles (1.3671, 4.3276) (1.1037, 4.0885) (0.3825, 3.8252) (-0.1443, 3.8252) knots 0 0 0 1 2 2 2
  spline S69 degree 2 poles (-0.1443, 3.8252) (-0.7034, 3.8292) (-1.5057, 4.0116) (-1.7691, 4.1291) knots 0 0 0 1 2 2 2
  line L139 (-1.7691, 4.1291) -> (-1.7691, 5.219)
  line L140 (-1.7691, 5.219) -> (-1.6556, 5.219)
  spline S70 degree 2 poles (-1.6556, 5.219) (-1.5584, 5.1663) (-1.3234, 5.0286) (-1.1329, 4.9556) knots 0 0 0 1 2 2 2
  spline S71 degree 2 poles (-1.1329, 4.9556) (-0.9547, 4.8868) (-0.5859, 4.7936) (-0.3631, 4.7936) knots 0 0 0 1 2 2 2
  spline S72 degree 2 poles (-0.3631, 4.7936) (-0.1686, 4.7936) (0.2852, 4.8908) (0.423, 5.0205) knots 0 0 0 1 2 2 2
  spline S73 degree 2 poles (0.423, 5.0205) (0.5243, 5.1218) (0.6377, 5.3689) (0.6377, 5.5756) knots 0 0 0 1 2 2 2
  spline S74 degree 2 poles (0.6377, 5.5756) (0.6377, 5.7539) (0.4919, 6.0051) (0.3744, 6.0821) knots 0 0 0 1 2 2 2
  spline S75 degree 2 poles (0.3744, 6.0821) (0.2042, 6.1955) (-0.282, 6.2603) (-0.4563, 6.2603) knots 0 0 0 1 2 2 2
  spline S76 degree 2 poles (-0.4563, 6.2603) (-0.7318, 6.2603) (-1.2545, 6.1712) (-1.4449, 6.1226) knots 0 0 0 1 2 2 2
  line L141 (-1.4449, 6.1226) -> (-1.5543, 6.1226)
  line L142 (-1.5543, 6.1226) -> (-1.5543, 8.9305)
  line L143 (-1.5543, 8.9305) -> (1.7601, 8.9305)
  line L144 (1.7601, 8.9305) -> (1.7601, 7.9864)
  line L145 (1.7601, 7.9864) -> (-0.3671, 7.9864)
  line L146 (-0.3671, 7.9864) -> (-0.3671, 7.1558)
  spline S77 degree 2 poles (-0.3671, 7.1558) (-0.2658, 7.1639) (0.0137, 7.172) (0.0907, 7.172) knots 0 0 0 1 2 2 2
  spline S78 degree 2 poles (0.0907, 7.172) (0.4513, 7.172) (1.0591, 7.0262) (1.2982, 6.8762) knots 0 0 0 1 2 2 2
  spline S79 degree 2 poles (1.2982, 6.8762) (1.5818, 6.6898) (1.8979, 6.0699) (1.8979, 5.6242) knots 0 0 0 1 2 2 2
  spline S80 degree 2 poles (15.852, 5.5391) (15.852, 4.749) (14.8512, 3.732) (13.976, 3.732) knots 0 0 0 1 2 2 2
  spline S81 degree 2 poles (13.976, 3.732) (13.5384, 3.732) (12.8536, 3.9832) (12.6146, 4.2304) knots 0 0 0 1 2 2 2
  spline S82 degree 2 poles (12.6146, 4.2304) (12.3309, 4.518) (12.0271, 5.4297) (12.0271, 6.0659) knots 0 0 0 1 2 2 2
  spline S83 degree 2 poles (12.0271, 6.0659) (12.0271, 6.7223) (12.3107, 7.7433) (12.6308, 8.1364) knots 0 0 0 1 2 2 2
  spline S84 degree 2 poles (12.6308, 8.1364) (12.9347, 8.5091) (13.9233, 8.9305) (14.6, 8.9305) knots 0 0 0 1 2 2 2
  spline S85 degree 2 poles (14.6, 8.9305) (14.8472, 8.9305) (15.3415, 8.8657) (15.4306, 8.8454) knots 0 0 0 1 2 2 2
  line L147 (15.4306, 8.8454) -> (15.4306, 7.8649)
  line L148 (15.4306, 7.8649) -> (15.3415, 7.8649)
  spline S86 degree 2 poles (15.3415, 7.8649) (15.2523, 7.9095) (14.8472, 8.0189) (14.5878, 8.0189) knots 0 0 0 1 2 2 2
  spline S87 degree 2 poles (14.5878, 8.0189) (14.0003, 8.0189) (13.3601, 7.3989) (13.2831, 6.8236) knots 0 0 0 1 2 2 2
  spline S88 degree 2 poles (13.2831, 6.8236) (13.5303, 6.9816) (14.0368, 7.168) (14.3569, 7.168) knots 0 0 0 1 2 2 2
  spline S89 degree 2 poles (14.3569, 7.168) (14.6284, 7.168) (15.1024, 7.0221) (15.2848, 6.8843) knots 0 0 0 1 2 2 2
  spline S90 degree 2 poles (15.2848, 6.8843) (15.5441, 6.6858) (15.852, 6.0415) (15.852, 5.5391) knots 0 0 0 1 2 2 2
  spline S91 degree 2 poles (14.3893, 4.7855) (14.4865, 4.907) (14.5919, 5.1907) (14.5919, 5.4783) knots 0 0 0 1 2 2 2
  spline S92 degree 2 poles (14.5919, 5.4783) (14.5919, 5.7215) (14.4703, 6.0375) (14.3609, 6.1307) knots 0 0 0 1 2 2 2
  spline S93 degree 2 poles (14.3609, 6.1307) (14.2475, 6.2279) (13.9679, 6.2968) (13.8099, 6.2968) knots 0 0 0 1 2 2 2
  spline S94 degree 2 poles (13.8099, 6.2968) (13.6762, 6.2968) (13.4006, 6.2279) (13.2791, 6.1793) knots 0 0 0 1 2 2 2
  spline S95 degree 2 poles (13.2791, 6.1793) (13.2791, 6.1469) (13.271, 5.9929) (13.271, 5.8754) knots 0 0 0 1 2 2 2
  spline S96 degree 2 poles (13.271, 5.8754) (13.271, 5.4419) (13.4209, 4.9192) (13.5384, 4.7855) knots 0 0 0 1 2 2 2
  spline S97 degree 2 poles (13.5384, 4.7855) (13.6235, 4.6761) (13.8504, 4.5829) (13.972, 4.5829) knots 0 0 0 1 2 2 2
  spline S98 degree 2 poles (13.972, 4.5829) (14.0732, 4.5829) (14.3083, 4.6842) (14.3893, 4.7855) knots 0 0 0 1 2 2 2
  spline S99 degree 2 poles (15.7548, 18.5991) (15.7548, 18.2303) (15.4833, 17.6266) (15.2199, 17.4159) knots 0 0 0 1 2 2 2
  spline S100 degree 2 poles (15.2199, 17.4159) (14.9566, 17.2052) (14.2394, 16.9783) (13.7248, 16.9783) knots 0 0 0 1 2 2 2
  spline S101 degree 2 poles (13.7248, 16.9783) (13.1413, 16.9783) (12.3066, 17.1728) (12.0433, 17.2944) knots 0 0 0 1 2 2 2
  line L149 (12.0433, 17.2944) -> (12.0433, 18.3803)
  line L150 (12.0433, 18.3803) -> (12.1648, 18.3803)
  spline S102 degree 2 poles (12.1648, 18.3803) (12.4403, 18.206) (13.1818, 17.9467) (13.4898, 17.9467) knots 0 0 0 1 2 2 2
  spline S103 degree 2 poles (13.4898, 17.9467) (13.6721, 17.9467) (14.0976, 18.0115) (14.2434, 18.1169) knots 0 0 0 1 2 2 2
  spline S104 degree 2 poles (14.2434, 18.1169) (14.3569, 18.202) (14.4946, 18.4491) (14.4946, 18.672) knots 0 0 0 1 2 2 2
  spline S105 degree 2 poles (14.4946, 18.672) (14.4946, 18.8948) (14.3002, 19.1339) (14.1381, 19.1906) knots 0 0 0 1 2 2 2
  spline S106 degree 2 poles (14.1381, 19.1906) (13.976, 19.2474) (13.5262, 19.2595) (13.352, 19.2595) knots 0 0 0 1 2 2 2
  line L151 (13.352, 19.2595) -> (13.1373, 19.2595)
  line L152 (13.1373, 19.2595) -> (13.1373, 20.1388)
  line L153 (13.1373, 20.1388) -> (13.3358, 20.1388)
  spline S107 degree 2 poles (13.3358, 20.1388) (13.5627, 20.1388) (13.9476, 20.1793) (14.0814, 20.2401) knots 0 0 0 1 2 2 2
  spline S108 degree 2 poles (14.0814, 20.2401) (14.2151, 20.3049) (14.365, 20.5318) (14.365, 20.7263) knots 0 0 0 1 2 2 2
  spline S109 degree 2 poles (14.365, 20.7263) (14.365, 20.8803) (14.2232, 21.0707) (14.1219, 21.1234) knots 0 0 0 1 2 2 2
  spline S110 degree 2 poles (14.1219, 21.1234) (14.0003, 21.1841) (13.6762, 21.2247) (13.5627, 21.2247) knots 0 0 0 1 2 2 2
  spline S111 degree 2 poles (13.5627, 21.2247) (13.3804, 21.2247) (12.9955, 21.1396) (12.8172, 21.0707) knots 0 0 0 1 2 2 2
  spline S112 degree 2 poles (12.8172, 21.0707) (12.6754, 21.018) (12.3674, 20.8478) (12.2945, 20.8033) knots 0 0 0 1 2 2 2
  line L154 (12.2945, 20.8033) -> (12.1891, 20.8033)
  line L155 (12.1891, 20.8033) -> (12.1891, 21.873)
  spline S113 degree 2 poles (12.1891, 21.873) (12.4485, 21.9824) (13.3237, 22.189) (13.7815, 22.189) knots 0 0 0 1 2 2 2
  spline S114 degree 2 poles (13.7815, 22.189) (14.2272, 22.189) (14.8836, 22.035) (15.1146, 21.8851) knots 0 0 0 1 2 2 2
  spline S115 degree 2 poles (15.1146, 21.8851) (15.3698, 21.7271) (15.6251, 21.2409) (15.6251, 20.937) knots 0 0 0 1 2 2 2
  spline S116 degree 2 poles (15.6251, 20.937) (15.6251, 20.5075) (15.1308, 19.8673) (14.7256, 19.7741) knots 0 0 0 1 2 2 2
  line L156 (14.7256, 19.7741) -> (14.7256, 19.7255)
  spline S117 degree 2 poles (14.7256, 19.7255) (14.9039, 19.7012) (15.2442, 19.5715) (15.4063, 19.4256) knots 0 0 0 1 2 2 2
  spline S118 degree 2 poles (15.4063, 19.4256) (15.5562, 19.296) (15.7548, 18.8827) (15.7548, 18.5991) knots 0 0 0 1 2 2 2
  dimension "d0" = 64
  dimension "d1" = 51
  dimension "d7" = 2
  dimension "d26" = 2.5
  dimension "d27" = 2.5
  dimension "d28" = 46
  dimension "d29" = 59
  constraints: 24 other
extrude "Extrusion8" cut sketch "Sketch11" against normal blind 0.1
body "Solid1"
